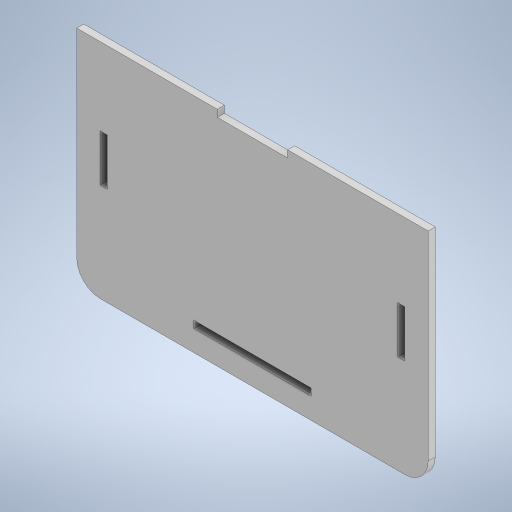
# Autodesk Inventor part: Cover
Saved by Autodesk Inventor 2023 (Build 270158000, 158)
## iProperties
Created: 2022-10-06
Part Number: Cover
Material: Generic
Document SubType Name: Modeling
Designer: digge
Density: 1 g/cm^3
Appearance: Default
Author: digge
Autodesk Inventor part; units mm, degrees
ref_plane "YZ Plane" through (0, 0, 0) normal (1, 0, 0) x (0, 1, 0)
ref_plane "XZ Plane" through (0, 0, 0) normal (0, 1, 0) x (-1, 0, 0)
ref_plane "XY Plane" through (0, 0, 0) normal (0, 0, 1) x (1, 0, 0)
sketch "Sketch1" plane through (0, 0, 0) normal (0, 0, 1) x (1, 0, 0)
  line L0 (-218.7343, 123.2169) -> (-218.7343, 28.2169)
  line L1 (-218.7343, 28.2169) -> (-68.7343, 28.2169)
  line L2 (-68.7343, 28.2169) -> (-68.7343, 123.2169)
  line L3 (-158.7343, 123.2169) -> (-158.7343, 120.2169)
  line L4 (-158.7343, 120.2169) -> (-128.7343, 120.2169)
  line L5 (-128.7343, 120.2169) -> (-128.7343, 123.2169)
  line L6 (-208.7343, 90.2169) -> (-205.7343, 90.2169)
  line L7 (-205.7343, 90.2169) -> (-205.7343, 70.2169)
  line L8 (-205.7343, 70.2169) -> (-208.7343, 70.2169)
  line L9 (-208.7343, 70.2169) -> (-208.7343, 90.2169)
  line L10 (-81.7343, 90.2169) -> (-78.7343, 90.2169)
  line L11 (-78.7343, 90.2169) -> (-78.7343, 70.2169)
  line L12 (-78.7343, 70.2169) -> (-81.7343, 70.2169)
  line L13 (-81.7343, 70.2169) -> (-81.7343, 90.2169)
  line L14 (-168.7343, 40.2169) -> (-118.7343, 40.2169)
  line L15 (-118.7343, 40.2169) -> (-118.7343, 37.2169)
  line L16 (-118.7343, 37.2169) -> (-168.7343, 37.2169)
  line L17 (-168.7343, 37.2169) -> (-168.7343, 40.2169)
  line L18 (-143.7343, 123.2169) -> (-143.7343, 28.2169) construction
  line L19 (-218.7343, 123.2169) -> (-158.7343, 123.2169)
  line L20 (-128.7343, 123.2169) -> (-68.7343, 123.2169)
  line L21 (-136.5327, 40.2169) -> (-136.5327, 120.2169) construction
  line L22 (-136.5327, 80.2169) -> (-68.7343, 80.2169) construction
  point P0 (0, 0)
  dimension "d0" = 150
  dimension "d1" = 95
  dimension "d3" = 3
  dimension "d4" = 3
  dimension "d5" = 3
  dimension "d6" = 20
  dimension "d7" = 10
  dimension "d8" = 10
  dimension "d9" = 30
  dimension "d10" = 3
  dimension "d11" = 9
  dimension "d12" = 50
  constraints: 46 end point, 9 perpendicular, 6 parallel, 5 horizontal, 5 point on line, 2 midpoint, 2 vertical, 3 other
  measures "d0" distance of L2.end L0.start
  measures "d1" distance of L1.end L2.end
  measures "d3" distance between parallel lines of L16 L14
  measures "d4" distance between parallel lines of L11 L13
  measures "d5" distance between parallel lines of L9 L7
  measures "d6" distance of L6.end L7.end
  measures "d7" distance between parallel lines of L0 L9
  measures "d8" distance between parallel lines of L2 L11
  measures "d9" distance of L5.end L3.start
  measures "d10" distance between parallel lines of L20 L4
  measures "d11" distance between parallel lines of L1 L16
  measures "d12" distance of L14.start L14.end
extrude "Extrusion1" add sketch "Sketch1" along normal blind 3
fillet "Fillet1" radius 10 2 edges at (-68.7343, 28.2169, 1.5) (-218.7343, 28.2169, 1.5)
body "Solid1"
